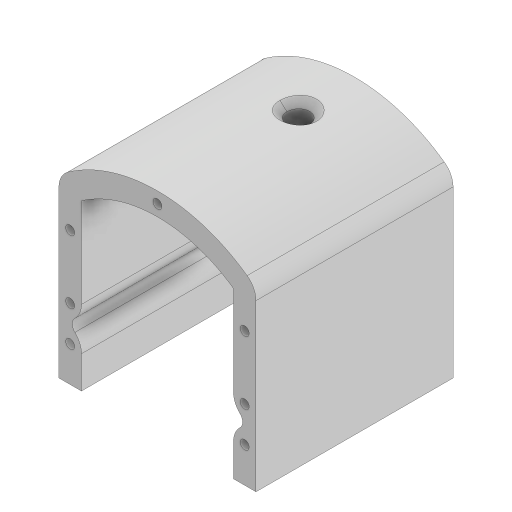
# Autodesk Inventor part: back wall
Saved by Autodesk Inventor 2024 (Build 280153000, 153)
## iProperties
Created: 2024-08-03
Part Number: back wall
Material: Generic
Document SubType Name: Modeling
Designer: chris
Density: 1 g/cm^3
Appearance: Default
Author: chris
Autodesk Inventor part; units mm, degrees
ref_plane "YZ Plane" through (0, 0, 0) normal (1, 0, 0) x (0, 1, 0)
ref_plane "XZ Plane" through (0, 0, 0) normal (0, 1, 0) x (-1, 0, 0)
ref_plane "XY Plane" through (0, 0, 0) normal (0, 0, 1) x (1, 0, 0)
sketch "Sketch1" plane through (0, 0, 0) normal (0, 0, 1) x (1, 0, 0)
  arc A0 (40.4395, 56.9532) -> (-40.4395, 56.9532) centre (0, 0) ccw
  arc A1 (-40.4395, 56.9532) -> (-44.45, 49.1869) centre (-34.925, 49.1869) ccw
  circle A2 centre (0, 64.77) radius 2
  arc A3 (44.45, 49.1869) -> (40.4395, 56.9532) centre (34.925, 49.1869) ccw
  line L0 (44.45, -25.4935) -> (44.45, 49.1869)
  line L1 (-44.45, 49.1869) -> (-44.45, -25.4935)
  circle A4 centre (-39.37, 34.8315) radius 2
  circle A5 centre (39.37, 34.8315) radius 2
  circle A6 centre (39.37, -9.6185) radius 2
  circle A7 centre (-39.37, -9.6185) radius 2
  circle A8 centre (-34.6, -1.2888) radius 2
  circle A9 centre (34.6, -1.2888) radius 2
  line L2 (-39.37, -9.6185) -> (-39.37, -25.4935)
  line L3 (-39.37, -25.4935) -> (-44.45, -25.4935)
  circle A10 centre (-34.6, -1.2888) radius 3.81
  circle A11 centre (34.6, -1.2888) radius 3.81
  line L4 (-34.29, -25.4935) -> (-34.29, 48.8579)
  arc A12 (34.29, 48.8579) -> (-34.29, 48.8579) centre (0, 0) ccw
  line L5 (34.29, 48.8579) -> (34.29, -25.4935)
  line L6 (-39.37, -25.4935) -> (-34.29, -25.4935)
  line L7 (34.29, -25.4935) -> (44.45, -25.4935)
  point P0 (0, 0)
  point P1 (-34.29, -5.0862)
  point P2 (-34.29, 2.5086)
  point P3 (34.29, 2.5086)
  point P4 (34.29, -5.0862)
  dimension "d0" = 7.62
  dimension "d1" = 7.62
  dimension "d2" = 10.16
  constraints: 16 end point, 13 centre point, 8 point on circle, 3 horizontal, 2 coincident, 1 vertical
  measures "d0" diameter of A10
  measures "d1" diameter of A11
  measures "d2" radial gap between concentric circles of A0 A12
extrude "Extrusion1" add sketch "Sketch1" along normal blind 88.9 contours A3 L0 L7 L5 A11 A12 L4 A10 L6 L3 L1 A1 A0 | A2 | A4
fillet "Fillet1" radius 9.525 4 edges at (-34.29, 2.5086, 44.45) (34.29, 2.5086, 44.45) (-34.29, -5.0862, 44.45) (34.29, -5.0862, 44.45)
sketch "Sketch5" plane through (34.29, -25.4935, 0) normal (0, -1, 0) x (1, 0, 0)
  line L0 (-68.58, 0) -> (-68.58, 88.9) projected
  line L1 (0, 88.9) -> (0, 0) projected
  line L2 (-68.58, 0) -> (0, 0)
  line L3 (-68.58, 0) -> (-34.29, 0)
  line L4 (-34.29, 0) -> (-34.29, 88.9)
  line L5 (-34.29, 0) -> (-34.29, 25.4)
  circle A0 centre (-34.29, 25.4) radius 5.08
  dimension "d39" = 25.4
  dimension "d40" = 10.16
  constraints: 8 end point, 1 centre point, 1 coincident, 1 collinear, 1 horizontal, 1 perpendicular, 1 point on line
  measures "d39" distance of L3.end L5.end
  measures "d40" diameter of A0
extrude "Extrusion5" cut sketch "Sketch5" against normal through all
sketch "Sketch6" plane through (0, 0, 0) normal (0, 0, -1) x (-1, 0, 0)
  arc A0 (-34.29, -10.9276) -> (-37.2329, -4.0427) centre (-43.815, -10.9276) ccw projected
  arc A1 (-37.2329, 1.4651) -> (-37.2329, -4.0427) centre (-34.6, -1.2888) ccw projected
  arc A2 (-37.2329, 1.4651) -> (-34.29, 8.35) centre (-43.815, 8.35) ccw projected
  line L0 (-34.29, 48.8579) -> (-34.29, 8.35) projected
  arc A3 (34.29, 48.8579) -> (-34.29, 48.8579) centre (0, 0) ccw projected
  line L1 (34.29, 8.35) -> (34.29, 48.8579) projected
  arc A4 (34.29, 8.35) -> (37.2329, 1.4651) centre (43.815, 8.35) ccw projected
  arc A5 (37.2329, -4.0427) -> (37.2329, 1.4651) centre (34.6, -1.2888) ccw projected
  arc A6 (37.2329, -4.0427) -> (34.29, -10.9276) centre (43.815, -10.9276) ccw projected
  line L2 (34.29, -25.4935) -> (34.29, -10.9276) projected
  line L3 (44.45, -25.4935) -> (34.29, -25.4935) projected
  line L4 (44.45, 49.1869) -> (44.45, -25.4935) projected
  arc A7 (44.45, 49.1869) -> (40.4395, 56.9532) centre (34.925, 49.1869) ccw projected
  arc A8 (40.4395, 56.9532) -> (-40.4395, 56.9532) centre (0, 0) ccw projected
  arc A9 (-40.4395, 56.9532) -> (-44.45, 49.1869) centre (-34.925, 49.1869) ccw projected
  line L5 (-44.45, -25.4935) -> (-44.45, 49.1869) projected
  line L6 (-34.29, -25.4935) -> (-44.45, -25.4935) projected
  line L7 (-34.29, -10.9276) -> (-34.29, -25.4935) projected
  circle A10 centre (39.37, -9.6185) radius 2 projected
  circle A11 centre (-39.37, -9.6185) radius 2 projected
  circle A12 centre (-39.37, 34.8315) radius 2 projected
  line L8 (39.37, 34.8315) -> (39.37, 42.769)
  line L9 (39.37, 42.769) -> (39.37, 26.894)
  line L10 (39.37, 42.769) -> (47.6019, 42.769)
  line L11 (39.37, 26.894) -> (47.6019, 26.894)
  line L12 (39.37, 42.769) -> (31.4554, 42.769)
  line L13 (39.37, 26.894) -> (31.1414, 26.894)
  point P0 (0, 0)
  point P1 (34.29, 42.769)
  point P2 (34.29, 26.894)
  point P3 (44.45, 26.894)
  point P4 (44.45, 42.769)
  dimension "d43" = 7.9375
  dimension "d44" = 15.875
  constraints: 12 end point, 4 horizontal, 1 point on line, 1 vertical
  measures "d43" distance of L8.start L8.end
  measures "d44" distance of L8.end L9.end
extrude "Extrusion6" cut sketch "Sketch6" against normal blind 10.16 contours L12 L8 L9 L13 L1 | L10 L4 L11 L9 L8
chamfer "Chamfer3" distance 3.175 angle 45 3 edges at (-44.45, 34.8315, 10.16) (-44.45, 42.769, 5.08) (-44.45, 26.894, 5.08)
chamfer "Chamfer4" distance 3.175 angle 45 1 edges at (-5.0799, 69.665, 25.4351)
sketch "Sketch7" plane through (0, 0, 88.9) normal (0, 0, 1) x (1, 0, 0)
  circle A0 centre (0, 64.77) radius 2 projected
  circle A1 centre (-39.37, 34.8315) radius 2 projected
  point P0 (0, 0)
extrude "Extrusion7" cut sketch "Sketch7" against normal blind 25.4
sketch "Sketch8" plane through (0, 0, 0) normal (0, 0, -1) x (-1, 0, 0)
  point P0 (0, 0)
extrude "Extrusion8" cut sketch "Sketch1" along normal blind 15.24 contours A2
sketch "Sketch9" plane through (0, 0, 88.9) normal (0, 0, 1) x (1, 0, 0)
  circle A0 centre (-39.37, 34.8315) radius 2 projected
  line L0 (-39.37, 34.8315) -> (-39.37, 6.2565)
  circle A1 centre (-39.37, 6.2565) radius 2
  circle A2 centre (39.37, 34.8315) radius 2 projected
  line L1 (39.37, 34.8315) -> (39.37, 6.2565)
  circle A3 centre (39.37, 6.2565) radius 2
  point P0 (0, 0)
  dimension "d57" = 28.575
  dimension "d58" = 4
  dimension "d59" = 28.575
  dimension "d60" = 4
  constraints: 4 end point, 2 centre point, 2 coincident, 2 vertical
  measures "d57" distance of L0.start L0.end
  measures "d58" diameter of A1
  measures "d59" distance of L1.start L1.end
  measures "d60" diameter of A3
extrude "Extrusion9" cut sketch "Sketch9" against normal blind 15.24 contours A1 | A3
body "Solid1"
